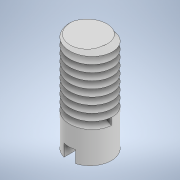
# Autodesk Inventor part: Винт 3x6
Saved by Autodesk Inventor 2020 (Build 240168000, 168)
## iProperties
Created: 2021-04-26
Part Number: Винт 3x6
Material: Типовые
Document SubType Name: Modeling
Designer: lbfas
Density: 1 g/cm^3
Appearance: По умолчанию
Author: lbfas
Autodesk Inventor part; units mm, degrees
ref_plane "YZ Plane" through (0, 0, 0) normal (1, 0, 0) x (0, 1, 0)
ref_plane "XZ Plane" through (0, 0, 0) normal (0, 1, 0) x (-1, 0, 0)
ref_plane "XY Plane" through (0, 0, 0) normal (0, 0, 1) x (1, 0, 0)
sketch "Эскиз1" plane through (0, 0, 0) normal (0, 1, 0) x (-1, 0, 0)
  circle A0 centre (0, 0) radius 1.75
  dimension "d0" = 3.5
  constraints: 1 centre point, 1 coincident
  measures "d0" diameter of A0
extrude "Выдавливание1" add sketch "Эскиз1" along normal blind 8
sketch "Эскиз3" plane through (0, 0, 0) normal (0, 0, 1) x (1, 0, 0)
  line L0 (1.75, 0) -> (-1.75, 0) projected
  line L1 (1.75, 2.7887) -> (1.25, 2.7887)
  line L2 (1.25, 2.7887) -> (1.75, 2.5)
  line L3 (1.75, 2.5) -> (1.75, 2.7887)
  line L4 (1.25, 2.7887) -> (1.75, 3.0774)
  line L5 (1.75, 2.7887) -> (1.75, 3.0774)
  line L6 (2, 2.5) -> (1.75, 2.5)
  line L7 (1.75, 0) -> (1.75, 8) projected
  point P0 (0, 0)
  dimension "d6" = 0.5
  dimension "d7" = 30
  constraints: 12 end point, 1 point on line, 1 symmetric about line
  measures "d6" distance of L1.start L1.end
  measures "d7" angle of L2 L1
coil "Пружина1" sketch "Эскиз3" operation cut axis through (0, 0, 0) along (0, 1, 0) pitch 0.577 turns 17.331023 hand left
sketch "Эскиз4" plane through (0, 0, 0) normal (0, -1, 0) x (1, 0, 0)
  line L0 (-0.4375, 0.2421) -> (-0.4375, -1.6944)
  circle A0 centre (0, 0) radius 1.75 projected
  line L1 (-0.4375, 0.2421) -> (-0.4375, 2.1786)
  line L2 (0.5, 0) -> (0.5, -1.9365)
  line L3 (0.5, 0) -> (0.5, 1.9365)
  point P0 (0.5, 1.6771)
  point P1 (-0.4375, 1.6944)
  point P2 (0.5, -1.6771)
  constraints: 8 end point, 2 other
extrude "Выдавливание3" cut sketch "Эскиз4" against normal blind 1 contours L1 A0 L3 L2 L0
